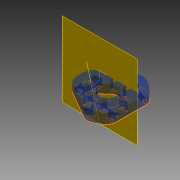
# Autodesk Inventor part: Platfrom_Top_14mm_Rev
Saved by Autodesk Inventor 2011 SP2 (Build 150309200, 309)
## iProperties
Created: 2011-03-08
Part Number: Platfrom_Top_14mm_Rev
Document SubType Name: Modeling
Designer: sungwook
Density: 1.38123 g/cm^3
Material: PET
Mass: 0.536789 g
Surface Area: 6.20753 cm^2
Volume: 0.388631 cm^3
Author: sungwook
Autodesk Inventor part; units mm, degrees
ref_plane "YZ Plane" through (0, 0, 0) normal (1, 0, 0) x (0, 1, 0)
ref_plane "XZ Plane" through (0, 0, 0) normal (0, 1, 0) x (-1, 0, 0)
ref_plane "XY Plane" through (0, 0, 0) normal (0, 0, 1) x (1, 0, 0)
sketch "Sketch1" plane through (0, 0, 0) normal (0, 0, 1) x (1, 0, 0)
  circle A0 centre (0, 0) radius 8.5
  dimension "d0" = 17
  constraints: 1 centre point, 1 coincident
  measures "d0" diameter of A0
extrude "Extrusion1" add sketch "Sketch1" along normal blind 3
sketch "Sketch2" plane through (0, 0, 0) normal (0, 0, -1) x (-1, 0, 0)
  circle A0 centre (0, 0) radius 8.5
  circle A1 centre (0, 0) radius 7
  line L0 (0, 0) -> (8.145676, 2.428571)
  line L1 (0, 0) -> (-1.969634, 8.268648)
  line L2 (11.9, 0) -> (-11.9, 0)
  circle A2 centre (-1.622051, 6.809475) radius 0.5
  circle A3 centre (6.708204, 2) radius 0.5
  dimension "d3" = 14
  dimension "d4" = 16.6015
  dimension "d5" = 86.7969
  dimension "d6" = 1
  dimension "d7" = 1
  dimension "d253" = 17
  dimension "d316" = 2.0066
  constraints: 4 end point, 4 point on circle, 3 centre point, 2 point on line, 1 coincident
  measures "d3" diameter of A1
  measures "d4" angle of L2 L0
  measures "d5" angle of L1 L0
  measures "d6" diameter of A2
  measures "d7" diameter of A3
  measures "d253" diameter of A0
hole "Mount Hole" at (0, 0, 0) direction (0, 0, 1) diameter 5.08 end through all
sketch "Sketch9" plane through (0, 0, 3) normal (0, 0, 1) x (1, 0, 0)
  circle A0 centre (0, 0) radius 8.5
  line L0 (6.5, 5.477226) -> (6.5, -5.477226)
  arc A1 (6.5, -5.477226) -> (6.5, 5.477226) centre (0, 0) ccw
  dimension "d85" = 10.95445
  dimension "d188" = 6.5
  constraints: 2 end point, 2 point on circle, 1 centre point, 1 coincident, 1 vertical, 2 other
  measures "d85" distance of L0.start L0.end
  measures "d188" distance from line of point (0, 0) L0
extrude "Extrusion4" cut sketch "Sketch9" against normal through all contours A0 L0 picked at (6.863527, 1.275107)
fillet "Fillet1" radius 2.5 2 edges at (6.5, 5.4772, 1.5) (6.5, -5.4772, 1.5)
pattern_circular "Circular Pattern6" count 3 over 360 about axis through (0, 0, -10) along (0, 0, 1) of "Extrusion4", "Fillet1"
sketch "Sketch14" plane through (6.5, -4.472136, 3) normal (1, 0, 0) x (0, 0, -1)
  line L0 (0, 0) -> (0, 8.944272)
  line L1 (6.084022, 4.472136) -> (-1.597337, 4.472136)
  line L2 (-0.5, 9.472136) -> (0.5, 9.472136)
  line L3 (0.5, 9.472136) -> (0.5, -0.527864)
  line L4 (0.5, -0.527864) -> (-0.5, -0.527864)
  line L5 (-0.5, -0.527864) -> (-0.5, 9.472136)
  point P0 (3, 4.472136)
  point P1 (-0.5, 4.472136)
  point P2 (0, 4.472136)
  dimension "d113" = 1
  dimension "d114" = 10
  dimension "d116" = 0.5
  constraints: 8 end point, 2 midpoint, 2 parallel, 1 horizontal, 1 horizontal alignment, 1 perpendicular
  measures "d113" distance of L2.start L2.end
  measures "d114" distance of L4.end L2.start
  measures "d116" distance between parallel lines of L3 L0
extrude "Extrusion7" cut sketch "Sketch14" against normal through all
sketch "Sketch15" plane through (6.5, -4.472136, 2.5) normal (0, 0, 1) x (1, 0, 0)
  ellipse E0 centre (-1.971593, -1.330533) end of major axis (-1.78835, -1.237005) minor radius 0.2 (-1.794972, -1.225083) -> (-2.143308, -1.225083) ccw
  line L0 (-0.056363, -0.527864) -> (-10.839746, -0.527864)
  arc A0 (-0.056363, -0.527864) -> (0, 0) centre (-2.5, 0) ccw
  line L1 (0, 8.944272) -> (0, 0)
  arc A1 (0, 8.944272) -> (-0.056363, 9.472136) centre (-2.5, 8.944272) ccw
  line L2 (-0.056363, 9.472136) -> (-10.839746, 9.472136)
  line L3 (-0.056363, 9.472136) -> (-10.839746, 9.472136)
  line L4 (-13.622983, 7.865233) -> (-10.839746, 9.472136)
  arc A2 (-13.622983, 7.865233) -> (-14.82006, 6.21185) centre (-12.372983, 5.70017) ccw
  arc A3 (-14.82006, 6.21185) -> (-14.82006, 2.732422) centre (-6.5, 4.472136) ccw
  arc A4 (-14.82006, 2.732422) -> (-13.622983, 1.079039) centre (-12.372983, 3.244102) ccw
  line L5 (-10.839746, -0.527864) -> (-13.622983, 1.079039)
  line L6 (-0.056363, -0.527864) -> (-10.839746, -0.527864)
  circle A5 centre (-8.492105, 1.017564) radius 0.5969
  circle A6 centre (-8.495694, 7.924636) radius 0.5969
  circle A7 centre (-2.512201, 4.474208) radius 0.5969
  circle A8 centre (-6.5, 4.472136) radius 2.54
  line L7 (-6.5, 4.472136) -> (-4.530366, 12.740784)
  circle A9 centre (-4.877949, 11.281611) radius 0.333327
  point P0 (-13.208204, 6.472136)
  point P1 (-13.208204, 6.472136)
  constraints: 2 coincident, 1 centre point, 3 other
ref_plane "Work Plane6" through (-6.708204, 2, 0) normal (-0.2857143, -0.9583148, 0) x (0.9583148, -0.2857143, 0)
ref_plane "Work Plane7" through (0, 0, 2.5) normal (0.9727821, -0.2317216, 0) x (0, 0, -1)
sketch "Sketch16" plane through (-6.708204, 2, 0) normal (-0.2857143, -0.9583148, 0) x (0.9583148, -0.2857143, 0)
  line L0 (7, 0) -> (-1.5, 0)
  line L1 (-0.5, 0) -> (0.5, 0)
  line L2 (0, 0) -> (14, 0)
  line L3 (0, 0) -> (-0.389585, -1.932124)
  dimension "d119" = 78.6
  constraints: 2 end point
  measures "d119" angle of L3 L0
hole "Hole7" at (-6.708204, 2, 0) direction (0.189418, -0.0564735, 0.9802712) diameter 0.5 end up to surface countersink diameter 1.5 countersink angle 90
sketch "Sketch24" plane through (-6.708204, 2, 0) normal (-0.2857143, -0.9583148, 0) x (0.9583148, -0.2857143, 0)
  line L0 (-0.735203, 0.148243) -> (-0.146239, 0.53955)
  line L1 (-0.735203, 0.148243) -> (0, 0)
  line L2 (-4.403947, 0) -> (18.403947, 0)
  line L3 (0.343896, 0.440721) -> (-0.146239, 0.53955)
  line L4 (-0.146239, 0.53955) -> (-1.273556, -0.209438)
  line L5 (-1.273556, -0.209438) -> (0, 0)
  line L6 (0.098829, 0.490136) -> (-0.146239, 0.53955)
  line L7 (0.098829, 0.490136) -> (0, 0)
  line L8 (-0.866397, -4.296848) -> (1.542608, 7.650481)
  point P0 (7, 0)
  constraints: 8 end point, 2 collinear, 1 midpoint, 1 perpendicular
revolve "Revolution5" cut sketch "Sketch24" angle 360 about axis through (-7.081549, 2.11131, -1.932124) along (0.189418, -0.0564735, 0.9802712) contours L1 L2 L4 | L5 L4 L2
sketch "Sketch18" plane through (0, 0, 2.5) normal (0.9727821, -0.2317216, 0) x (0, 0, -1)
  line L0 (2.5, -7) -> (2.5, 7)
  line L1 (2.5, 0) -> (2.5, 8.5)
  line L2 (2.5, 7) -> (3.587465, 7.219271)
  dimension "d130" = 78.6
  constraints: 2 end point
  measures "d130" angle of L2 L1
hole "Hole8" at (1.622051, 6.809475, 0) direction (-0.0458015, -0.1922775, 0.9802712) diameter 0.5 end through all countersink diameter 1.5 countersink angle 90
sketch "Sketch19" plane through (0, 0, 2.5) normal (0.9727821, -0.2317216, 0) x (0, 0, -1)
  line L0 (2.059279, 6.656104) -> (1.96045, 7.146239)
  line L1 (1.96045, 7.146239) -> (2.351757, 7.735203)
  line L2 (1.96045, 7.146239) -> (2.87511, 8.522913)
  line L3 (-5.403717, 5.406331) -> (6.636934, 7.834152)
  line L4 (1.96045, 7.146239) -> (2.5, 7)
  line L5 (2.87511, 8.522913) -> (2.5, 7)
  point P0 (2.5, 0)
  constraints: 6 end point, 1 collinear, 1 point on line
revolve "Revolution4" cut sketch "Sketch19" angle 360 about axis through (1.622051, 6.809475, 0) along (0.0458015, 0.1922775, -0.9802712) contours L1 L2 L5 L4
pattern_circular "Circular Pattern8" count 3 over 360 about axis through (0, 0, -10) along (0, 0, 1) of "Hole7", "Hole8", "Revolution4", "Revolution5"
sketch "Sketch29" plane through (0, 0, 0) normal (0, 0, -1) x (-1, 0, 0)
  arc A0 (-5.666667, -6.335526) -> (-2.653393, -8.07524) centre (0, 0) ccw
  constraints: 1 coincident
hole "Spring Slot" [suppressed]
sketch "Sketch30" plane through (0, 0, 0) normal (0, 0, -1) x (-1, 0, 0)
  circle A0 centre (2.286, 0) radius 1.016
  circle A1 centre (0, 0) radius 2.54 projected
  dimension "d213" = 2.032
  dimension "d256" = 2.286
  constraints: 1 centre point
  measures "d213" diameter of A0
  measures "d256" distance of A0.centre A1.centre
hole "Jig Slot" at (-2.286, 0, 0) direction (0, 0, 1) diameter 2.032 end through all
sketch "Sketch40" plane through (0, 0, 0) normal (0, 1, 0) x (-1, 0, 0)
  line L0 (-2.54, 0) -> (-6.5, 0)
  line L1 (-6.5, 0) -> (-6.5, 2.5)
  line L2 (-6.5, 2.5) -> (-2.54, 2.5)
  line L3 (-2.54, 2.5) -> (-2.54, 0)
  line L4 (3.302, 2.5) -> (8.5, 2.5)
  line L5 (8.5, 2.5) -> (8.5, 0)
  line L6 (8.5, 0) -> (3.302, 0)
  line L7 (5.310514, 2.5) -> (4.242285, -1.486685)
  line L8 (3.302, 0) -> (3.302, 2.5)
  point P0 (0, 0)
  point P1 (-5.334, 2)
  point P2 (0, 2)
  point P3 (4.776399, 0.506657)
  dimension "d245" = 5.334
  dimension "d246" = 5.334
  dimension "d247" = 105
  constraints: 2 end point, 1 midpoint, 1 point on line
  measures "d245" distance of L7.start point (0, 2)
  measures "d246" distance of point (0, 2) point (-5.334, 2)
  measures "d247" angle of L4 L7
ref_plane "Work Plane12" through (-5.310514, 0, 2.5) normal (-0.258819, 0, 0.9659258) x (0, -1, 0)
sketch "Sketch51" plane through (-5.310514, 0, 2.5) normal (-0.258819, 0, 0.9659258) x (0, -1, 0)
  ellipse E0 centre (1.870864, -0.998581) end of major axis (1.835152, -0.722436) minor radius 0.25
  ellipse E1 centre (-1.870864, -0.998581) end of major axis (-1.835152, -0.722436) minor radius 0.25
  line L0 (-5, 1.931852) -> (-5, 1.005013)
  line L1 (-5, 1.005013) -> (-5.516877, 1.931852)
  line L2 (-5.516877, 1.931852) -> (-5, 1.931852)
  line L3 (5, 1.005013) -> (5, 1.931852)
  line L4 (5, 1.931852) -> (5.516877, 1.931852)
  line L5 (5.516877, 1.931852) -> (5, 1.005013)
  ellipse E2 centre (1.228034, -0.582311) end of major axis (1.228034, -3.170502) minor radius 2.5 (1.739714, -3.115711) -> (3.393097, -1.876407) ccw
  ellipse E3 centre (0, 5.497848) end of major axis (0, -3.301999) minor radius 8.5 (-1.739714, -3.115711) -> (1.739714, -3.115711) ccw
  ellipse E4 centre (-1.228034, -0.582311) end of major axis (-1.228034, -3.170502) minor radius 2.5 (-3.393097, -1.876407) -> (-1.739714, -3.115711) ccw
  line L6 (-3.393097, -1.876407) -> (-4.439527, 0)
  line L7 (-4.439527, 0) -> (4.439527, 0)
  line L8 (4.439527, 0) -> (3.393097, -1.876407)
  line L9 (-2.5, 0.762) -> (2.5, 0.762)
  line L10 (2.5, 0.762) -> (2.5, 0)
  line L11 (2.5, 0) -> (-2.5, 0)
  line L12 (-2.5, 0) -> (-2.5, 0.762)
  point P0 (0, 4.482515)
  point P1 (0, 0.762)
  dimension "d249" = 0.762
  dimension "d250" = 5
  constraints: 8 end point, 2 parallel, 1 horizontal, 1 midpoint, 1 perpendicular, 1 point on line, 1 vertical alignment, 5 other
  measures "d249" distance between parallel lines of L11 L9
  measures "d250" distance between parallel lines of L10 L12
extrude "Extrusion15" [suppressed]
sketch "Sketch58" plane through (0, 0, 0) normal (0, 0, -1) x (-1, 0, 0)
  arc A0 (-5.666667, -6.335526) -> (-2.653393, -8.07524) centre (0, 0) ccw
  circle A1 centre (0, 0) radius 3.9878
  line L0 (11.9, 0) -> (-11.9, 0)
  point P0 (-3.9878, 0)
  dimension "d277" = 7.9756
  constraints: 1 coincident, 1 horizontal alignment, 1 point on line, 2 other
hole "Hole17" at (3.9878, 0, 0) direction (0, 0, 1) diameter 1.1938 end through all
pattern_circular "Circular Pattern11" count 3 over 360 about axis through (0, 0, -10) along (0, 0, 1) of "Hole17"
sketch "Sketch59" plane through (0, 0, 0) normal (0, 0, -1) x (-1, 0, 0)
  line L0 (11.9, 0) -> (-11.9, 0)
  arc A0 (8.32006, -1.739714) -> (8.32006, 1.739714) centre (0, 0) ccw
  point P0 (-5.2324, 0)
  dimension "d311" = 5.2324
  constraints: 1 point on line
  measures "d311" distance of A0.centre point (-5.232, 0)
hole "Hole18" at (5.2324, 0, 0) direction (0, 0, 1) diameter 0.4318 end through all
sketch "Sketch60" plane through (0, 0, 0) normal (0, 0, -1) x (-1, 0, 0)
  circle A0 centre (-5.2324, 0) radius 0.2159
  circle A1 centre (1.9939, -3.453536) radius 0.5969
  circle A2 centre (1.9939, 3.453536) radius 0.5969
  circle A3 centre (-3.9878, 0) radius 0.5969
  line L0 (4.009221, -2.5) -> (4.009221, 2.5)
  line L1 (4.009221, 2.5) -> (4.798102, 2.5)
  line L2 (4.798102, 2.5) -> (4.798102, -2.5)
  line L3 (4.798102, -2.5) -> (4.009221, -2.5)
  ellipse E0 centre (-5.202995, 4.919961) end of major axis (-4.623523, 4.372011) minor radius 0.765728
  ellipse E1 centre (-5.202995, -4.919961) end of major axis (-4.623523, -4.372011) minor radius 0.765728
  ellipse E2 centre (-1.659314, -6.965906) end of major axis (-1.474511, -6.190094) minor radius 0.765728
  ellipse E3 centre (6.862309, -2.045945) end of major axis (6.098034, -1.818083) minor radius 0.765728
  ellipse E4 centre (6.862309, 2.045945) end of major axis (6.098034, 1.818083) minor radius 0.765728
  circle A4 centre (0, 0) radius 2.54
  arc A5 (7.122983, -3.393097) -> (8.32006, -1.739714) centre (5.872983, -1.228034) ccw
  arc A6 (8.32006, -1.739714) -> (8.32006, 1.739714) centre (0, 0) ccw
  arc A7 (8.32006, 1.739714) -> (7.122983, 3.393097) centre (5.872983, 1.228034) ccw
  line L4 (7.122983, 3.393097) -> (-0.622983, 7.865233)
  arc A8 (-0.622983, 7.865233) -> (-2.653393, 8.07524) centre (-1.872983, 5.70017) ccw
  arc A9 (-2.653393, 8.07524) -> (-5.666667, 6.335526) centre (0, 0) ccw
  arc A10 (-5.666667, 6.335526) -> (-6.5, 4.472136) centre (-4, 4.472136) ccw
  line L5 (-6.5, 4.472136) -> (-6.5, -4.472136)
  arc A11 (-6.5, -4.472136) -> (-5.666667, -6.335526) centre (-4, -4.472136) ccw
  arc A12 (-5.666667, -6.335526) -> (-2.653393, -8.07524) centre (0, 0) ccw
  arc A13 (-2.653393, -8.07524) -> (-0.622983, -7.865233) centre (-1.872983, -5.70017) ccw
  line L6 (-0.622983, -7.865233) -> (7.122983, -3.393097)
  ellipse E5 centre (-1.659314, 6.965906) end of major axis (-1.474511, 6.190094) minor radius 0.765728
  dimension "d296" = 0.4318
  dimension "d297" = 5.2324
  constraints: 6 other
  measures "d297" distance of A0.centre A4.centre
pattern_circular "Circular Pattern12" count 3 over 360 about axis through (0, 0, -10) along (0, 0, 1) of "Hole18"
sketch "Sketch62" plane through (6.5, -4.472136, 2.5) normal (0, 0, 1) x (1, 0, 0)
  arc A0 (-8.828333, 3.457018) -> (-8.828333, 5.487254) centre (-6.5, 4.472136) ccw
  arc A1 (-14.82006, 6.21185) -> (-14.82006, 2.732422) centre (-6.5, 4.472136) ccw
  line L0 (-11.7578, 7.012136) -> (-10.9958, 7.012136)
  line L1 (-10.9958, 7.012136) -> (-10.9958, 1.932136)
  line L2 (-10.9958, 1.932136) -> (-11.7578, 1.932136)
  line L3 (-11.7578, 1.932136) -> (-11.7578, 7.012136)
  point P0 (-10.9958, 4.472136)
  dimension "d302" = 0.762
  dimension "d303" = 5.08
  dimension "d304" = 4.4958
  constraints: 8 end point, 2 parallel, 1 horizontal, 1 horizontal alignment, 1 midpoint, 1 perpendicular
  measures "d302" distance between parallel lines of L1 L3
  measures "d303" distance of L1.end L0.end
  measures "d304" distance from line of A0.centre L1
extrude "Extrusion16" cut sketch "Sketch62" against normal through all
sketch "Sketch65" plane through (6.5, -4.472136, 2.5) normal (0, 0, 1) x (1, 0, 0)
  arc A0 (-8.828333, 3.457018) -> (-8.828333, 5.487254) centre (-6.5, 4.472136) ccw
  line L0 (-18.041641, 4.472136) -> (3.249845, 4.472136)
  point P0 (-10.31, 4.472136)
  point P1 (-4.595, 1.172579)
  point P2 (-4.595, 7.771693)
  dimension "d317" = 3.81
  dimension "d320" = 360
  constraints: 1 point on line, 4 other
  measures "d317" distance of A0.centre point (-10.31, 4.472)
hole "Hole19" at (1.905, -3.299557, 2.5) at (1.905, 3.299557, 2.5) direction (0, 0, -1) diameter 1.4732 end through all
sketch "Sketch66" plane through (0.622983, -7.865233, 0) normal (-0.5, -0.8660254, 0) x (0.8660254, -0.5, 0)
  line L0 (-8.944272, 0) -> (-8.944272, 2.5)
  line L1 (-8.944272, 2.5) -> (-8.944272, 0)
  point P0 (-4.472136, 0)
  point P1 (-8.944272, 1.25)
  constraints: 2 end point, 1 collinear, 1 midpoint
hole "Hole20" [suppressed]
sketch "Sketch71" plane through (0, 0, 0) normal (0, 0, -1) x (-1, 0, 0)
  circle A0 centre (-1.905, 3.299557) radius 0.7366
  circle A1 centre (-1.905, -3.299557) radius 0.7366
  line L0 (5.2578, 2.54) -> (5.2578, -2.54)
  line L1 (5.2578, -2.54) -> (4.4958, -2.54)
  line L2 (4.4958, -2.54) -> (4.4958, 2.54)
  line L3 (4.4958, 2.54) -> (5.2578, 2.54)
  circle A2 centre (2.6162, -4.531391) radius 0.2159
  circle A3 centre (2.6162, 4.531391) radius 0.2159
  circle A4 centre (-5.2324, 0) radius 0.2159
  circle A5 centre (1.9939, -3.453536) radius 0.5969
  circle A6 centre (1.9939, 3.453536) radius 0.5969
  circle A7 centre (-3.9878, 0) radius 0.5969
  ellipse E0 centre (-1.659314, 6.965906) end of major axis (-1.474511, 6.190094) minor radius 0.765728
  arc A8 (7.122983, -3.393097) -> (8.32006, -1.739714) centre (5.872983, -1.228034) ccw
  arc A9 (8.32006, -1.739714) -> (8.32006, 1.739714) centre (0, 0) ccw
  arc A10 (8.32006, 1.739714) -> (7.122983, 3.393097) centre (5.872983, 1.228034) ccw
  line L4 (7.122983, 3.393097) -> (-0.622983, 7.865233)
  arc A11 (-0.622983, 7.865233) -> (-2.653393, 8.07524) centre (-1.872983, 5.70017) ccw
  arc A12 (-2.653393, 8.07524) -> (-5.666667, 6.335526) centre (0, 0) ccw
  arc A13 (-5.666667, 6.335526) -> (-6.5, 4.472136) centre (-4, 4.472136) ccw
  line L5 (-6.5, 4.472136) -> (-6.5, -4.472136)
  arc A14 (-6.5, -4.472136) -> (-5.666667, -6.335526) centre (-4, -4.472136) ccw
  arc A15 (-5.666667, -6.335526) -> (-2.653393, -8.07524) centre (0, 0) ccw
  arc A16 (-2.653393, -8.07524) -> (-0.622983, -7.865233) centre (-1.872983, -5.70017) ccw
  line L6 (-0.622983, -7.865233) -> (7.122983, -3.393097)
  arc A17 (2.328333, -1.015118) -> (2.328333, 1.015118) centre (2.286, 0) ccw
  arc A18 (2.328333, 1.015118) -> (2.328333, -1.015118) centre (0, 0) ccw
  ellipse E1 centre (6.862309, 2.045945) end of major axis (6.098034, 1.818083) minor radius 0.765728
  ellipse E2 centre (6.862309, -2.045945) end of major axis (6.098034, -1.818083) minor radius 0.765728
  ellipse E3 centre (-1.659314, -6.965906) end of major axis (-1.474511, -6.190094) minor radius 0.765728
  ellipse E4 centre (-5.202995, -4.919961) end of major axis (-4.623523, -4.372011) minor radius 0.765728
  ellipse E5 centre (-5.202995, 4.919961) end of major axis (-4.623523, 4.372011) minor radius 0.765728
  ellipse E6 centre (6.613495, 1.971763) end of major axis (6.542066, 2.211342) minor radius 0.245068
  ellipse E7 centre (6.225129, 1.855975) end of major axis (6.469529, 1.928841) minor radius 0.25
  ellipse E8 centre (6.613495, 1.971763) end of major axis (6.542066, 2.211342) minor radius 0.245068
  line L7 (6.225129, 1.855975) -> (6.613495, 1.971763)
  line L8 (6.419312, 1.913869) -> (6.419312, 5.492757)
  point P0 (6.419312, 3.799362)
  constraints: 4 end point, 2 point on line, 1 midpoint, 1 parallel, 10 other
ref_plane "Work Plane15" through (-6.419312, 3.799362, 0) normal (0, 1, 0) x (-1, 0, 0)
sketch "Sketch72" plane through (-6.419312, 3.799362, 0) normal (0, 1, 0) x (-1, 0, 0)
  line L0 (0, 0) -> (0, 2.5)
  line L1 (0.703672, 2.5) -> (-2.079566, 2.5)
  point P0 (-6.419312, 0)
  point P1 (0, 1.25)
  constraints: 2 end point, 1 midpoint, 1 point on line
hole "Hole24" at (-6.419312, 3.799362, 1.25) direction (0, -1, 0) diameter 1.1938 depth 2.032
hole "Hole25" at (-6.419312, 3.799362, 1.25) direction (0, 1, 0) diameter 1.1938 end through all
mirror "Mirror2" about plane through (0, 0, 0) normal (0, 1, 0) of "Hole24", "Hole25"
pattern_circular "Circular Pattern14" [suppressed]
pattern_circular "Circular Pattern15" count 3 over 360 about axis through (0, 0, -10) along (0, 0, 1) of "Hole24", "Hole25", "Mirror2"
equation "\"d3\" = topD"
equation "\"d4\" = topTh0"
equation "\"d5\" = topTh1"
equation "\"baseInitD\" = 4"
equation "\"baseTh0\" = 48.463041deg"
equation "\"baseTh1\" = 23.073918deg"
equation "\"topInitD\" = 4"
equation "\"topTh0\" = 16.6015deg"
equation "\"topTh1\" = 86.7969deg"
equation "\"dFlexure\" = 0.38"
equation "\"lFlexure\" = 1.5"
equation "\"topD\" = 14"
equation "\"dMotor\" = 1.44"
equation "\"springBaseD\" = 8"
equation "\"springTopD\" = 8"
equation "\"springInitL\" = 12.7"
equation "\"lMotor\" = 22.35"
equation "\"topH\" = 21.66629"
equation "\"springL\" = 30.86629"
equation "\"springLset\" = 3.5"
equation "\"springDeform\" = 18.16629"
equation "\"springUnderCut\" = 9.2"
equation "\"springLO\" = 33.86629"
equation "\"lFlexureOffset\" = 1.95"
equation "\"dM2Y\" = 7.00349"
equation "\"dM2X\" = -1.34133"
equation "\"dM1X\" = 6.73587"
equation "\"dM1Y\" = 2.34012"
equation "\"dM1Xt\" = 6.59227"
equation "\"dM1Yt\" = -0.43704"
equation "\"dM2Xt\" = -3.67462"
equation "\"dM2Yt\" = 5.49055"
equation "\"d46\" = 14"
equation "\"d47\" = 16.354015deg"
equation "\"d48\" = 87.29197deg"
equation "\"GuideRod\" = 2"
equation "\"baseOD\" = 23"
equation "\"CSpringOD\" = 5.537"
equation "\"CSpringCD\" = 0.254"
equation "\"GuideTubingOD\" = 4"
equation "\"GuideTubingID\" = 2"
equation "\"CSpringID\" = 5.029"
equation "\"lOCTprobe\" = 1905"
equation "\"OCToffset\" = 365.252"
equation "\"lOCT\" = 1473.2"
equation "\"lOCTprobeNorm\" = 1838.452"
equation "\"lOCTprobeNom\" = 1838.452"
equation "\"OCTd0\" = 508"
equation "\"OCTd1\" = 254"
body "Solid1"
